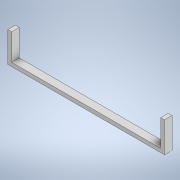
# Autodesk Inventor part: tester7.75
Saved by Autodesk Inventor 2020.2 (Build 242310000, 310)
## iProperties
Created: 2020-02-21
Part Number: tester7.75
Material: Generic
Document SubType Name: Modeling
Designer: ColinP
Density: 1 g/cm^3
Appearance: Default
Author: ColinP
Autodesk Inventor part; units mm, degrees
ref_plane "YZ Plane" through (0, 0, 0) normal (1, 0, 0) x (0, 1, 0)
ref_plane "XZ Plane" through (0, 0, 0) normal (0, 1, 0) x (-1, 0, 0)
ref_plane "XY Plane" through (0, 0, 0) normal (0, 0, 1) x (1, 0, 0)
sketch "Sketch1" plane through (0, 0, 0) normal (0, 1, 0) x (-1, 0, 0)
  line L0 (4.4017, 8.3575) -> (-0.5983, 8.3575)
  line L1 (-0.5983, 8.3575) -> (-0.5983, -1.6425)
  line L2 (-0.5983, -1.6425) -> (4.4017, -1.6425)
  line L3 (4.4017, -1.6425) -> (4.4017, 8.3575)
  point P0 (0, 0)
  dimension "d0" = 5
  dimension "d1" = 10
  constraints: 8 end point, 2 parallel, 1 horizontal, 1 perpendicular
  measures "d0" distance of L2.end L1.end
  measures "d1" distance of L1.end L0.end
extrude "Extrusion1" add sketch "Sketch1" along normal blind 40
sketch "Sketch2" plane through (0.5983, 0, 8.3575) normal (1, 0, 0) x (0, 0, -1)
  line L0 (10, 0) -> (0, 0) projected
  line L1 (0, 0) -> (10, 0)
  line L2 (10, 0) -> (10, 5)
  line L3 (10, 5) -> (0, 5)
  line L4 (0, 5) -> (0, 0)
  point P0 (8.3575, 0)
  dimension "d4" = 5
  constraints: 8 end point, 2 parallel, 1 horizontal, 1 perpendicular
  measures "d4" distance of L2.end L1.end
extrude "Extrusion2" add sketch "Sketch2" along normal blind 201.85
sketch "Sketch3" plane through (202.4483, 0, 8.3575) normal (1, 0, 0) x (0, 0, -1)
  point P0 (8.3575, 0)
sketch "Sketch4" plane through (0.5983, 5, 8.3575) normal (0, 1, 0) x (1, 0, 0)
  line L0 (-5, 0) -> (201.85, 0) projected
  line L1 (-5, 10) -> (201.85, 10) projected
  line L2 (201.85, 0) -> (196.85, 0)
  line L3 (196.85, 0) -> (196.85, 10)
  line L4 (196.85, 10) -> (201.85, 10)
  line L5 (201.85, 10) -> (201.85, 0)
  point P0 (-0.5983, 8.3575)
  point P1 (196.85, 0)
  dimension "d7" = 5
  constraints: 8 end point, 2 parallel, 1 horizontal, 1 perpendicular, 1 point on line
  measures "d7" distance of L3.end L4.end
extrude "Extrusion3" add sketch "Sketch4" along normal blind 35
body "Solid1"
